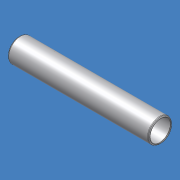
# Autodesk Inventor part: 04R-4.75650C
Saved by Autodesk Inventor 2012 (Build 160160000, 160)
## iProperties
Category: PARTsolutions
Created: 2013-01-20
Part Number: 04R-4.75650C
Catalog Web Link: www.cadenas.de
Description: Tube - Original Line - Standard Air Cylinders
Document SubType Name: Modeling
Designer: PARTsolutions
Material: Default
Density: 1 g/cm^3
Mass: 4.49995 g
Surface Area: 153.859 cm^2
Volume: 4.49995 cm^3
NB: 04R-4.75650C
NN: Tube
NT: Original Line - Standard Air Cylinders
NBSYN: $PN.
LINA: 04R-4.75650C
PN: 04R-4.75650C
BORE: 0.75000000
BOREPN: 04
MNTALG: '' , 'Front Nose' , 'BF' , 'Front Block' , 'BFT' , 'Front Trunnion' , 'A' , 'Adjustable Stroke'
ACTING: R
ACTINGALG: '' , 'Single Acting' , 'R' , 'Reverse/Double Acting'
NRALG: '' , 'N/A'
L: 4.7565
OD: 0.8075
ODN: 0.8050
ODP: 0.8625
ODB: 0.8325
ID: 0.7615
DV: 0.00000000
LV: 0.00000000
LV1: 0.00000000
G: 0.0300
FOURHOLES: 0
AA: 0.3750
BB: 0.0940
SR: C
SRALG: 'C' , 'Carbon Steel Rod' , 'SR' , '303 Stainless Steel Rod' , '' , '303 Stainless Steel Rod'
KT: DUMMY
SUPPLIER: Bimba
ARTICLENO: 04R-4.75650C
BOMINFO: 04R-4.75650C
CREATOR: CADENAS GmbH
PSOL_IDENT_0: {\\10.0.0.242\data_v9\23d-libs\bimba\bimba\bimba_imperial\bimba_full_line\original_line_cylinders\st
PSOL_IDENT_1: andard_air_cylinders\tube.prj},192 {VTYP=3D},{NB=04R-4.75650C},{LINA=04R-4.75650C},{NN=Tube},{DATE=2
PSOL_IDENT_2: 0.08.2011 07:16:50},{GEOMDATE=18.02.2011 00:00:00},{VERSION=},{LINEID=40},{LINESUBID=-1},{WBVAR=MNT,
PSOL_IDENT_3: ACTING,NR,L,FOURHOLES,SR}  {NB=04R-4.75650C},{LINA=04R-4.75650C},{KT=DUMMY},{PN=04R-4.75650C},{BORE=
PSOL_IDENT_4: 0.75000000},{BOREPN=04},{MNT=},{MNTALG='' , 'Front Nose' , 'BF' , 'Front Block' , 'BFT' , 'Front Tru
PSOL_IDENT_5: nnion' , 'A' , 'Adjustable Stroke'},{ACTING=R},{ACTINGALG= '' , 'Single Acting' , 'R' , 'Reverse/Dou
PSOL_IDENT_6: ble Acting' },{NR=},{NRALG= '' , 'N/A' },{L=4.7565},{OD=0.8075},{ODN=0.8050},{ODP=0.8625},{ODB=0.832
PSOL_IDENT_7: 5},{ID=0.7615},{DV=0.00000000},{LV=0.00000000},{LV1=0.00000000},{G=0.0300},{FOURHOLES=0},{AA=0.3750}
PSOL_IDENT_8: ,{BB=0.0940},{SR=C},{SRALG= 'C' , 'Carbon Steel Rod' , 'SR' , '303 Stainless Steel Rod' , '' , '303
PSOL_IDENT_9: Stainless Steel Rod'}
Title: 04R-4.75650C
Author: Cadenas PARTsolutions
Comments: Original Line - Standard Air Cylinders
Autodesk Inventor part; units mm, degrees
sketch "Sketch_1" plane through (0, 0, 0) normal (0, 0, 1) x (1, 0, 0)
  line L0 (120.8151, 0) -> (0, 0)
  arc A0 (-0.6395, 9.3472) -> (-0.6395, 9.1676) centre (-0.5497, 9.2574) ccw
  line L1 (-0.6395, 9.1676) -> (-0.381, 8.9091)
  line L2 (-0.381, 8.9091) -> (0, 8.9091)
  line L3 (0, 8.9091) -> (0.762, 9.671)
  line L4 (0.762, 9.671) -> (120.0531, 9.671)
  line L5 (120.0531, 9.671) -> (120.8151, 8.9091)
  line L6 (120.8151, 8.9091) -> (121.1961, 8.9091)
  line L7 (121.1961, 8.9091) -> (121.4546, 9.1676)
  arc A1 (121.4546, 9.1676) -> (121.4546, 9.3472) centre (121.3648, 9.2574) ccw
  line L8 (121.4546, 9.3472) -> (120.7697, 10.0321)
  arc A2 (120.7697, 10.0321) -> (120.2309, 10.2553) centre (120.2309, 9.4933) ccw
  line L9 (120.2309, 10.2553) -> (0.5842, 10.2553)
  arc A3 (0.5842, 10.2553) -> (0.0454, 10.0321) centre (0.5842, 9.4933) ccw
  line L10 (0.0454, 10.0321) -> (-0.6395, 9.3472)
  constraints: 22 end point, 8 point on circle, 4 centre point
revolve "Revolution1" add sketch "Sketch_1" angle 360 about axis through (120.8151, 0, 0) along (1, 0, 0)
ref_plane "tube_front_XY" through (0, 0, 0) normal (1, 0, 0) x (0, 0, -1)
ref_plane "tube_front_YZ" through (0, 0, 0) normal (0, 0, -1) x (0, 1, 0)
ref_plane "tube_front_ZX" through (0, 0, 0) normal (0, 1, 0) x (1, 0, 0)
ref_plane "tube_rear_XY" through (120.8151, 0, 0) normal (1, 0, 0) x (0, 0, -1)
ref_plane "tube_rear_YZ" through (120.8151, 0, 0) normal (0, 0, -1) x (0, 1, 0)
ref_plane "tube_rear_ZX" through (120.8151, 0, 0) normal (0, 1, 0) x (1, 0, 0)
ref_plane "cp1_XY" through (60.4076, 10.2553, 0) normal (1, 0, 0) x (0, 0, -1)
ref_plane "cp1_YZ" through (60.4076, 10.2553, 0) normal (0, 0, -1) x (0, 1, 0)
ref_plane "cp1_ZX" through (60.4076, 10.2553, 0) normal (0, 1, 0) x (1, 0, 0)
ref_plane "cp2_XY" through (60.4076, 0, -10.2553) normal (1, 0, 0) x (0, 0, -1)
ref_plane "cp2_YZ" through (60.4076, 0, -10.2553) normal (0, 0, -1) x (0, 1, 0)
ref_plane "cp2_ZX" through (60.4076, 0, -10.2553) normal (0, 1, 0) x (1, 0, 0)
ref_plane "cp3_XY" through (60.4076, -10.2553, 0) normal (1, 0, 0) x (0, 0, -1)
ref_plane "cp3_YZ" through (60.4076, -10.2553, 0) normal (0, 0, -1) x (0, 1, 0)
ref_plane "cp3_ZX" through (60.4076, -10.2553, 0) normal (0, 1, 0) x (1, 0, 0)
ref_plane "cp4_XY" through (60.4076, 0, 10.2553) normal (1, 0, 0) x (0, 0, -1)
ref_plane "cp4_YZ" through (60.4076, 0, 10.2553) normal (0, 0, -1) x (0, 1, 0)
ref_plane "cp4_ZX" through (60.4076, 0, 10.2553) normal (0, 1, 0) x (1, 0, 0)
body "Solid1"
